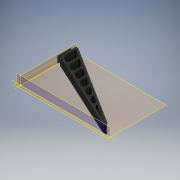
# Autodesk Inventor part: leg
Saved by Autodesk Inventor 2017 (Build 210142000, 142)
## iProperties
Created: 2020-06-17
Part Number: leg
Material: ABS Plastic
Document SubType Name: Modeling
Designer: HAYNIE R&D
Density: 1.06 g/cm^3
Appearance: Glossy - Black
Author: HAYNIE R&D
Autodesk Inventor part; units mm, degrees
sketch "Sketch1" plane through (0, 0, 0) normal (0, 0, 1) x (1, 0, 0)
  line L0 (0, 113.4196) -> (0, 163.4196)
  line L1 (0, 163.4196) -> (5, 163.4196)
  line L2 (5, 163.4196) -> (256, 5.04)
  line L3 (256, 5.04) -> (256, 0.0001)
  line L4 (256, 0.0001) -> (246, 0.0001)
  line L5 (256, 0.0001) -> (266, 0.0001) construction
  line L6 (246, 0.0001) -> (0, 113.4196)
  dimension "d1" = 50
  dimension "d2" = 163.4196
  dimension "d5" = 5
  dimension "d14" = 10
  dimension "d15" = 180
  constraints: 14 end point, 3 horizontal, 2 vertical, 1 collinear
  measures "d1" distance of L0.start L0.end
  measures "d2" vertical distance of L3.end L0.end
  measures "d5" distance of L0.end L1.end
  measures "d14" distance of L3.end L4.end
  measures "d15" angle of L4 L5
extrude "Extrusion1" add sketch "Sketch1" along normal blind 25
shell "Shell3" thickness 5 removed faces 2 at (83.6667, 92.2798, 25) at (83.6667, 92.2798, 0)
sketch "Sketch4" plane through (0, 0, 25) normal (0, 0, 1) x (1, 0, 0)
  line L0 (30, 141.7326) -> (30, 105.0938)
  line L1 (245.599, 5.6908) -> (5, 116.6202) projected
  line L2 (35, 102.7885) -> (35, 138.5776)
  line L3 (5, 157.5075) -> (245.599, 5.6908) projected
  line L4 (30, 105.0938) -> (35, 102.7885)
  line L5 (30, 141.7326) -> (35, 138.5776)
  line L6 (5, 116.6202) -> (5, 157.5075) projected
  line L7 (60, 122.8028) -> (60, 91.2622)
  line L8 (65, 119.6478) -> (65, 88.9569)
  line L9 (60, 122.8028) -> (65, 119.6478)
  line L10 (60, 91.2622) -> (65, 88.9569)
  line L11 (90, 103.8729) -> (90, 77.4305)
  line L12 (95, 100.7179) -> (95, 75.1252)
  line L13 (90, 103.8729) -> (95, 100.7179)
  line L14 (90, 77.4305) -> (95, 75.1252)
  line L15 (120, 84.9431) -> (120, 63.5989)
  line L16 (125, 81.7881) -> (125, 61.2936)
  line L17 (120, 84.9431) -> (125, 81.7881)
  line L18 (120, 63.5989) -> (125, 61.2936)
  line L19 (150, 66.0132) -> (150, 49.7672)
  line L20 (155, 62.8583) -> (155, 47.4619)
  line L21 (149.9292, 66.0579) -> (155, 62.8583)
  line L22 (150, 49.7672) -> (155, 47.4619)
  line L23 (180, 47.0834) -> (180, 35.9355)
  line L24 (185, 43.9284) -> (185, 33.6303)
  line L25 (180, 47.0834) -> (185, 43.9284)
  line L26 (180, 35.9355) -> (185, 33.6303)
  point P0 (0, 0)
  dimension "d22" = 25
  dimension "d23" = 5
  dimension "d26" = 25
  dimension "d28" = 5
  dimension "d31" = 25
  dimension "d32" = 5
  dimension "d33" = 25
  dimension "d34" = 5
  dimension "d35" = 25
  dimension "d36" = 5
  dimension "d37" = 25
  dimension "d38" = 5
  constraints: 48 end point, 10 vertical, 1 point on line, 28 other
  measures "d22" distance between parallel lines of L0 L6
  measures "d23" distance between parallel lines of L2 L0
  measures "d26" distance between parallel lines of L7 L2
  measures "d28" distance between parallel lines of L8 L7
  measures "d31" distance between parallel lines of L11 L8
  measures "d32" distance between parallel lines of L12 L11
  measures "d33" distance between parallel lines of L15 L12
  measures "d34" distance between parallel lines of L16 L15
  measures "d35" distance between parallel lines of L19 L16
  measures "d36" distance between parallel lines of L20 L19
  measures "d37" distance between parallel lines of L23 L20
  measures "d38" distance between parallel lines of L24 L23
extrude "Extrusion4" add sketch "Sketch4" against normal blind 25 contours L3 L2 L1 L0 | L3 L8 L1 L7 | L3 L12 L1 L11 | L3 L16 L1 L15 | L19 L3 L20 L1 | L23 L3 L24 L1
chamfer "Chamfer1" distance 5 angle 45 1 edges at (256, 5.04, 12.5)
fillet "Fillet1" radius 20 1 edges at (5, 163.4196, 12.5)
fillet "Fillet2" radius 20 1 edges at (251.7714, 7.7082, 12.5)
chamfer "Chamfer3" distance 5 angle 45 6 edges at (35, 102.7885, 12.5) (65, 88.9569, 12.5) (95, 75.1252, 12.5) (125, 61.2936, 12.5) (155, 47.4619, 12.5) (185, 33.6303, 12.5)
chamfer "Chamfer4" distance 5 angle 45 7 edges at (30, 105.0938, 12.5) (60, 91.2622, 12.5) (90, 77.4305, 12.5) (120, 63.5989, 12.5) (150, 49.7672, 12.5) (180, 35.9355, 12.5) (245.599, 5.6908, 12.5)
chamfer "Chamfer5" distance 5 angle 45 6 edges at (30, 141.7326, 12.5) (60, 122.8028, 12.5) (90, 103.8729, 12.5) (120, 84.9431, 12.5) (150, 66.0132, 12.5) (180, 47.0834, 12.5)
chamfer "Chamfer6" distance 5 angle 45 7 edges at (5, 157.5075, 12.5) (35, 138.5776, 12.5) (65, 119.6478, 12.5) (95, 100.7179, 12.5) (125, 81.7881, 12.5) (155, 62.8583, 12.5) (185, 43.9284, 12.5)
chamfer "Chamfer7" distance 5 angle 45 1 edges at (5, 116.6202, 12.5)
sketch "Sketch5" plane through (0, 113.4196, 0) normal (-1, 0, 0) x (0, 0, 1)
  line L0 (26.875, 1.25) -> (36.25, 1.25) construction
  line L1 (7.5, -0.0169) -> (17.5, -0.0169)
  line L2 (17.5, -0.0169) -> (17.5, 24.9831)
  line L3 (17.5, 24.9831) -> (7.5, 24.9831)
  line L4 (7.5, 24.9831) -> (7.5, -0.0169)
  line L5 (0, 0) -> (0, 50) projected
  line L6 (25, 50) -> (25, 0) projected
  point P0 (0, -113.4196)
  dimension "d67" = 25
  dimension "d70" = 7.5
  dimension "d71" = 7.5
  dimension "d72" = 10
  constraints: 10 end point, 2 horizontal, 2 parallel, 1 perpendicular
  measures "d67" distance of L2.end L1.end
  measures "d70" distance between parallel lines of L5 L4
  measures "d71" distance between parallel lines of L6 L2
  measures "d72" distance between parallel lines of L2 L4
extrude "Extrusion5" add sketch "Sketch5" along normal blind 5.25
sketch "Sketch7" plane through (-5.25, 113.4196, 0) normal (-1, 0, 0) x (0, 0, 1)
  line L0 (17.5, 0) -> (25, 0) projected
  line L1 (3, 40) -> (22, 40)
  line L2 (22, 40) -> (22, 0)
  line L3 (22, 0) -> (3, 0)
  line L4 (3, 0) -> (3, 40)
  line L5 (25, 50) -> (25, 0) projected
  line L6 (0, 0) -> (0, 50) projected
  point P0 (0, -113.4196)
  dimension "d73" = 3
  dimension "d74" = 3
  dimension "d75" = 19
  dimension "d76" = 40
  constraints: 8 end point, 2 parallel, 1 horizontal, 1 perpendicular, 1 point on line
  measures "d73" distance between parallel lines of L5 L2
  measures "d74" distance between parallel lines of L4 L6
  measures "d75" distance between parallel lines of L2 L4
  measures "d76" distance of L2.end L1.end
extrude "Extrusion6" add sketch "Sketch7" along normal blind 2.5
move or copy body "Move Body1" bodies to move or copy 1 copy no translate (7.75, 0, 0)
body "Solid1"
